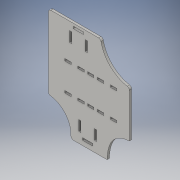
# Autodesk Inventor part: Part4
Saved by Autodesk Inventor 2016 (Build 200138000, 138)
## iProperties
Created: 2017-10-02
Part Number: Part4
Material: Generic
Document SubType Name: Modeling
Designer: student
Density: 1 g/cm^3
Appearance: Default
Author: student
Autodesk Inventor part; units mm, degrees
ref_plane "YZ Plane" through (0, 0, 0) normal (1, 0, 0) x (0, 1, 0)
ref_plane "XZ Plane" through (0, 0, 0) normal (0, 1, 0) x (-1, 0, 0)
ref_plane "XY Plane" through (0, 0, 0) normal (0, 0, 1) x (1, 0, 0)
sketch "Sketch1" plane through (0, 0, 0) normal (0, 0, 1) x (1, 0, 0)
  line L0 (8.2438, 0) -> (0, 0) construction
  line L1 (8.2438, 0) -> (8.2438, 2.921) construction
  line L2 (0, 2.921) -> (8.2438, 2.921) construction
  line L3 (0, 0) -> (0, 2.921) construction
  line L4 (24.6043, 0) -> (16.297, 0) construction
  line L5 (24.6043, 0) -> (24.6043, 2.921) construction
  line L6 (16.297, 2.921) -> (24.6043, 2.921) construction
  line L7 (16.297, 0) -> (16.297, 2.921) construction
  line L8 (36.8746, 0) -> (28.5674, 0) construction
  line L9 (36.8746, 0) -> (36.8746, 2.921) construction
  line L10 (28.5674, 2.921) -> (36.8746, 2.921) construction
  line L11 (28.5674, 0) -> (28.5674, 2.921) construction
  line L12 (49.145, 0) -> (40.8378, 0) construction
  line L13 (49.145, 0) -> (49.145, 2.921) construction
  line L14 (40.8378, 2.921) -> (49.145, 2.921) construction
  line L15 (40.8378, 0) -> (40.8378, 2.921) construction
  line L16 (65.442, 0) -> (57.1983, 0) construction
  line L17 (65.442, 0) -> (65.442, 2.921) construction
  line L18 (57.1983, 2.921) -> (65.442, 2.921) construction
  line L19 (57.1983, 0) -> (57.1983, 2.921) construction
  line L20 (65.442, -34.798) -> (57.1983, -34.798) construction
  line L21 (65.442, -34.798) -> (65.442, -31.877) construction
  line L22 (57.1983, -31.877) -> (65.442, -31.877) construction
  line L23 (57.1983, -34.798) -> (57.1983, -31.877) construction
  line L24 (49.145, -34.798) -> (40.8378, -34.798) construction
  line L25 (49.145, -34.798) -> (49.145, -31.877) construction
  line L26 (40.8378, -31.877) -> (49.145, -31.877) construction
  line L27 (40.8378, -34.798) -> (40.8378, -31.877) construction
  line L28 (36.8746, -34.798) -> (28.5674, -34.798) construction
  line L29 (36.8746, -34.798) -> (36.8746, -31.877) construction
  line L30 (28.5674, -31.877) -> (36.8746, -31.877) construction
  line L31 (28.5674, -34.798) -> (28.5674, -31.877) construction
  line L32 (24.6043, -34.798) -> (16.297, -34.798) construction
  line L33 (24.6043, -34.798) -> (24.6043, -31.877) construction
  line L34 (16.297, -31.877) -> (24.6043, -31.877) construction
  line L35 (16.297, -34.798) -> (16.297, -31.877) construction
  line L36 (8.2438, -34.798) -> (0, -34.798) construction
  line L37 (8.2438, -34.798) -> (8.2438, -31.877) construction
  line L38 (0, -31.877) -> (8.2438, -31.877) construction
  line L39 (0, -34.798) -> (0, -31.877) construction
  line L40 (0.1849, 0.127) -> (8.0589, 0.127)
  line L41 (8.0589, 0.127) -> (8.0589, 2.794)
  line L42 (8.0589, 2.794) -> (0.1849, 2.794)
  line L43 (0.1849, 2.794) -> (0.1849, 0.127)
  line L44 (0.1849, 0.127) -> (8.0589, 2.794) construction
  line L45 (8.0589, 0.127) -> (0.1849, 2.794) construction
  line L46 (16.5136, 0.127) -> (24.3876, 0.127)
  line L47 (24.3876, 0.127) -> (24.3876, 2.794)
  line L48 (24.3876, 2.794) -> (16.5136, 2.794)
  line L49 (16.5136, 2.794) -> (16.5136, 0.127)
  line L50 (28.784, 0.127) -> (36.658, 0.127)
  line L51 (36.658, 0.127) -> (36.658, 2.794)
  line L52 (36.658, 2.794) -> (28.784, 2.794)
  line L53 (28.784, 2.794) -> (28.784, 0.127)
  line L54 (41.0544, 0.127) -> (48.9284, 0.127)
  line L55 (48.9284, 0.127) -> (48.9284, 2.794)
  line L56 (48.9284, 2.794) -> (41.0544, 2.794)
  line L57 (41.0544, 2.794) -> (41.0544, 0.127)
  line L58 (57.3832, 0.127) -> (65.2572, 0.127)
  line L59 (65.2572, 0.127) -> (65.2572, 2.794)
  line L60 (65.2572, 2.794) -> (57.3832, 2.794)
  line L61 (57.3832, 2.794) -> (57.3832, 0.127)
  line L62 (0.1849, -34.671) -> (8.0589, -34.671)
  line L63 (8.0589, -34.671) -> (8.0589, -32.004)
  line L64 (8.0589, -32.004) -> (0.1849, -32.004)
  line L65 (0.1849, -32.004) -> (0.1849, -34.671)
  line L66 (16.5136, -34.671) -> (24.3876, -34.671)
  line L67 (24.3876, -34.671) -> (24.3876, -32.004)
  line L68 (24.3876, -32.004) -> (16.5136, -32.004)
  line L69 (16.5136, -32.004) -> (16.5136, -34.671)
  line L70 (28.784, -34.671) -> (36.658, -34.671)
  line L71 (36.658, -34.671) -> (36.658, -32.004)
  line L72 (36.658, -32.004) -> (28.784, -32.004)
  line L73 (28.784, -32.004) -> (28.784, -34.671)
  line L74 (41.0544, -34.671) -> (48.9284, -34.671)
  line L75 (48.9284, -34.671) -> (48.9284, -32.004)
  line L76 (48.9284, -32.004) -> (41.0544, -32.004)
  line L77 (41.0544, -32.004) -> (41.0544, -34.671)
  line L78 (57.3832, -34.671) -> (65.2572, -34.671)
  line L79 (65.2572, -34.671) -> (65.2572, -32.004)
  line L80 (65.2572, -32.004) -> (57.3832, -32.004)
  line L81 (57.3832, -32.004) -> (57.3832, -34.671)
  line L82 (10.7417, 40.386) -> (23.7211, 40.386) construction
  line L83 (23.7211, 40.386) -> (23.7211, 43.307) construction
  line L84 (10.7417, 43.307) -> (23.7211, 43.307) construction
  line L85 (10.7417, 40.386) -> (10.7417, 43.307) construction
  line L86 (5.8589, 36.1433) -> (5.8589, 23.1639) construction
  line L87 (5.8589, 23.1639) -> (8.7799, 23.1639) construction
  line L88 (8.7799, 36.1433) -> (8.7799, 23.1639) construction
  line L89 (5.8589, 36.1433) -> (8.7799, 36.1433) construction
  line L90 (25.6828, 36.1433) -> (25.6828, 23.1639) construction
  line L91 (25.6828, 23.1639) -> (28.6038, 23.1639) construction
  line L92 (28.6038, 36.1433) -> (28.6038, 23.1639) construction
  line L93 (25.6828, 36.1433) -> (28.6038, 36.1433) construction
  line L94 (17.3905, -54.5598) -> (17.3905, -67.5392) construction
  line L95 (17.3905, -67.5392) -> (20.3115, -67.5392) construction
  line L96 (20.3115, -54.5598) -> (20.3115, -67.5392) construction
  line L97 (17.3905, -54.5598) -> (20.3115, -54.5598) construction
  line L98 (37.0112, -54.5598) -> (37.0112, -67.5392) construction
  line L99 (37.0112, -67.5392) -> (39.9322, -67.5392) construction
  line L100 (39.9322, -54.5598) -> (39.9322, -67.5392) construction
  line L101 (37.0112, -54.5598) -> (39.9322, -54.5598) construction
  line L102 (22.1717, -74.9317) -> (35.1511, -74.9317) construction
  line L103 (35.1511, -74.9317) -> (35.1511, -72.0107) construction
  line L104 (22.1717, -72.0107) -> (35.1511, -72.0107) construction
  line L105 (22.1717, -74.9317) -> (22.1717, -72.0107) construction
  line L106 (6.0113, 23.3163) -> (6.0113, 35.9909)
  line L107 (6.0113, 35.9909) -> (8.7799, 35.9909)
  line L108 (8.7799, 35.9909) -> (8.7799, 23.3163)
  line L109 (8.7799, 23.3163) -> (6.0113, 23.3163)
  line L110 (6.0113, 23.3163) -> (8.7799, 35.9909) construction
  line L111 (6.0113, 35.9909) -> (8.7799, 23.3163) construction
  line L112 (25.6828, 23.3163) -> (25.6828, 35.9909)
  line L113 (25.6828, 35.9909) -> (28.4514, 35.9909)
  line L114 (28.4514, 35.9909) -> (28.4514, 23.3163)
  line L115 (28.4514, 23.3163) -> (25.6828, 23.3163)
  line L116 (17.4667, -67.5138) -> (17.4667, -54.8392)
  line L117 (17.4667, -54.8392) -> (20.2353, -54.8392)
  line L118 (20.2353, -54.8392) -> (20.2353, -67.5138)
  line L119 (20.2353, -67.5138) -> (17.4667, -67.5138)
  line L120 (37.0874, -67.5138) -> (37.0874, -54.8392)
  line L121 (37.0874, -54.8392) -> (39.856, -54.8392)
  line L122 (39.856, -54.8392) -> (39.856, -67.5138)
  line L123 (39.856, -67.5138) -> (37.0874, -67.5138)
  line L124 (28.6614, -72.0107) -> (28.6614, -74.9317) construction
  line L125 (22.3241, -74.8555) -> (34.9987, -74.8555)
  line L126 (34.9987, -74.8555) -> (34.9987, -72.0869)
  line L127 (34.9987, -72.0869) -> (22.3241, -72.0869)
  line L128 (22.3241, -72.0869) -> (22.3241, -74.8555)
  line L129 (22.3241, -74.8555) -> (34.9987, -72.0869) construction
  line L130 (34.9987, -74.8555) -> (22.3241, -72.0869) construction
  line L131 (17.2314, 40.386) -> (17.2314, 43.307) construction
  line L132 (10.8941, 40.4622) -> (23.5687, 40.4622)
  line L133 (23.5687, 40.4622) -> (23.5687, 43.2308)
  line L134 (23.5687, 43.2308) -> (10.8941, 43.2308)
  line L135 (10.8941, 43.2308) -> (10.8941, 40.4622)
  line L136 (10.8941, 40.4622) -> (23.5687, 43.2308) construction
  line L137 (23.5687, 40.4622) -> (10.8941, 43.2308) construction
  line L138 (-17.4388, 46.3259) -> (42.3239, 46.3259)
  line L139 (80.9862, 8.6137) -> (80.9862, -46.4509)
  line L140 (53.0791, -80.6741) -> (10.9143, -80.6741)
  line L141 (-20.6138, -43.5391) -> (-20.6138, 43.1509)
  arc A0 (45.433, 43.7942) -> (78.3699, 11.7391) centre (85.5855, 52.1022) ccw
  arc A1 (7.7429, -77.3488) -> (-17.857, -46.6864) centre (-21.7455, -75.9507) ccw
  spline S0 degree 2 poles (80.9862, -46.4509) (53.9185, -48.0993) (53.0791, -80.6741) knots 0 0 0 1 1 1
  arc A2 (-17.4388, 46.3259) -> (-20.6138, 43.1509) centre (-17.4388, 43.1509) ccw
  arc A3 (45.433, 43.7942) -> (42.3239, 46.3259) centre (42.3239, 43.1509) ccw
  arc A4 (80.9862, 8.6137) -> (78.3699, 11.7391) centre (77.8112, 8.6137) ccw
  arc A5 (7.7429, -77.3488) -> (10.9143, -80.6741) centre (10.9143, -77.4991) ccw
  arc A6 (-20.6138, -43.5391) -> (-17.857, -46.6864) centre (-17.4388, -43.5391) ccw
  point P0 (4.1219, 1.4605)
  point P1 (20.4506, 1.4605)
  point P2 (32.721, 1.4605)
  point P3 (44.9914, 1.4605)
  point P4 (61.3202, 1.4605)
  point P5 (4.1219, -33.3375)
  point P6 (20.4506, -33.3375)
  point P7 (32.721, -33.3375)
  point P8 (44.9914, -33.3375)
  point P9 (61.3202, -33.3375)
  point P10 (7.3956, 29.6536)
  point P11 (27.0671, 29.6536)
  point P12 (18.851, -61.1765)
  point P13 (38.4717, -61.1765)
  point P14 (28.6614, -73.4712)
  point P15 (17.2314, 41.8465)
  point P16 (-20.6138, 46.3259)
  point P17 (44.9914, 46.3259)
  point P18 (7.3956, -80.6741)
  point P19 (61.3281, -54.8411)
  point P20 (-20.6138, -46.4509)
  point P21 (80.9862, 11.358)
  dimension "d0" = 7.874
  dimension "d1" = 2.667
  dimension "d2" = 7.874
  dimension "d3" = 2.667
  dimension "d4" = 7.874
  dimension "d5" = 2.667
  dimension "d6" = 7.874
  dimension "d7" = 2.667
  dimension "d8" = 7.874
  dimension "d9" = 2.667
  dimension "d10" = 7.874
  dimension "d11" = 2.667
  dimension "d12" = 7.874
  dimension "d13" = 2.667
  dimension "d14" = 7.874
  dimension "d15" = 2.667
  dimension "d16" = 7.874
  dimension "d17" = 2.667
  dimension "d18" = 7.874
  dimension "d19" = 2.667
  dimension "d20" = 12.6746
  dimension "d21" = 2.7686
  dimension "d22" = 12.6746
  dimension "d23" = 2.7686
  dimension "d24" = 12.6746
  dimension "d25" = 2.7686
  dimension "d26" = 12.6746
  dimension "d27" = 2.7686
  dimension "d28" = 12.6746
  dimension "d29" = 2.7686
  dimension "d30" = 12.6746
  dimension "d31" = 2.7686
  dimension "d36" = 3.175
  dimension "d37" = 3.175
  dimension "d38" = 3.175
  constraints: 156 end point, 35 parallel, 19 perpendicular, 18 point on circle, 14 midpoint, 11 horizontal, 10 tangent, 7 centre point, 6 point on line, 2 equal radius, 5 other
  measures "d0" distance of L40.start L40.end
  measures "d1" distance of L41.end L40.end
  measures "d2" distance of L46.start L46.end
  measures "d3" distance of L48.start L46.end
  measures "d4" distance of L50.start L50.end
  measures "d5" distance of L52.start L50.end
  measures "d6" distance of L54.start L54.end
  measures "d7" distance of L56.start L54.end
  measures "d8" distance of L58.start L58.end
  measures "d9" distance of L60.start L58.end
  measures "d10" distance of L62.start L62.end
  measures "d11" distance of L64.start L62.end
  measures "d12" distance of L66.start L66.end
  measures "d13" distance of L68.start L66.end
  measures "d14" distance of L70.start L70.end
  measures "d15" distance of L72.start L70.end
  measures "d16" distance of L74.start L74.end
  measures "d17" distance of L76.start L74.end
  measures "d18" distance of L78.start L78.end
  measures "d19" distance of L80.start L78.end
  measures "d20" distance of L106.start L106.end
  measures "d21" distance of L106.end L107.end
  measures "d22" distance of L112.start L113.start
  measures "d23" distance of L113.start L113.end
  measures "d24" distance of L116.start L117.start
  measures "d25" distance of L117.start L117.end
  measures "d26" distance of L120.start L121.start
  measures "d27" distance of L121.start L121.end
  measures "d28" distance of L125.start L125.end
  measures "d29" distance of L126.end L125.end
  measures "d30" distance of L132.start L132.end
  measures "d31" distance of L133.end L132.end
  measures "d36" radius of A2
  measures "d37" radius of A5
  measures "d38" radius of A6
extrude "Extrusion1" add sketch "Sketch1" against normal blind 2.921
body "Solid1"
